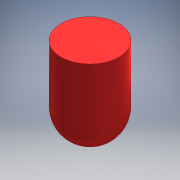
# Autodesk Inventor part: Toggle_LED
Saved by Autodesk Inventor 2016 (Build 200138000, 138)
## iProperties
Created: 2016-04-13
Part Number: Toggle_LED
Material: Polycarbonate, Clear
Document SubType Name: Modeling
Designer: agmle
Density: 1.2 g/cm^3
Appearance: Light Red
Author: agmle
Autodesk Inventor part; units mm, degrees
ref_plane "YZ Plane" through (0, 0, 0) normal (1, 0, 0) x (0, 1, 0)
ref_plane "XZ Plane" through (0, 0, 0) normal (0, 1, 0) x (-1, 0, 0)
ref_plane "XY Plane" through (0, 0, 0) normal (0, 0, 1) x (1, 0, 0)
sketch "Sketch1" plane through (0, 0, 0) normal (0, 1, 0) x (-1, 0, 0)
  arc A0 (0, -1.35) -> (1.35, 0) centre (0, 0) ccw
  line L0 (0, 2.65) -> (1.35, 2.65)
  line L1 (1.35, 2.65) -> (1.35, 0)
  line L2 (0, 2.65) -> (0, -1.35)
  dimension "d0" = 2.7
  dimension "d1" = 4
  constraints: 6 end point, 2 point on circle, 1 centre point, 1 coincident, 1 point on line, 1 tangent
  measures "d0" diameter of A0
revolve "Revolution1" add sketch "Sketch1" angle 360 about axis through (0, 0, 2.65) along (0, 0, -1)
body "Solid1"
